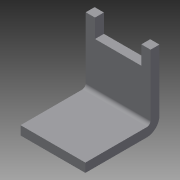
# Autodesk Inventor part: Glider
Saved by Autodesk Inventor 2013 (Build 170138000, 138)
## iProperties
Created: 2013-01-31
Part Number: Glider
Material: Generic
Document SubType Name: Sheet Metal
Designer: actoennies
Density: 1 g/cm^3
Sheet Metal Rule: Default
Author: actoennies
Autodesk Inventor part; units mm, degrees
ref_plane "YZ Plane" through (0, 0, 0) normal (1, 0, 0) x (0, 1, 0)
ref_plane "XZ Plane" through (0, 0, 0) normal (0, 1, 0) x (-1, 0, 0)
ref_plane "XY Plane" through (0, 0, 0) normal (0, 0, 1) x (1, 0, 0)
sketch "Sketch1" plane through (0, 0, 0) normal (0, 0, 1) x (1, 0, 0)
  line L0 (0, 0) -> (0, 6.35)
  line L1 (0, 6.35) -> (-3.175, 6.35)
  line L2 (-3.175, 6.35) -> (-3.175, -3.175)
  line L3 (0, 0) -> (15.875, 0)
  line L4 (15.875, 0) -> (15.875, 6.35)
  line L5 (15.875, 6.35) -> (19.05, 6.35)
  line L6 (19.05, 6.35) -> (19.05, -3.175)
  line L7 (-3.175, -3.175) -> (-3.175, -19.05)
  line L8 (-3.175, -19.05) -> (19.05, -19.05)
  line L9 (19.05, -19.05) -> (19.05, -3.175)
  dimension "d0" = 6.35
  dimension "d1" = 3.175
  dimension "d2" = 9.525
  dimension "d3" = 15.875
  dimension "d4" = 3.175
  dimension "d6" = 15.875
  measures "d0" distance of L0.start L0.end
  measures "d1" distance of L0.end L1.end
  measures "d2" distance of L1.end L2.end
  measures "d3" distance of L0.start L3.end
  measures "d4" distance of L4.end L5.end
  measures "d6" distance of L2.end L7.end
extrude "Plate1" add sketch "Sketch1" along normal blind 3.048
sketch "Sketch2" plane through (19.05, -16.002, 0) normal (0, -1, 0) x (1, 0, 0)
  line L0 (-22.225, 0) -> (0, 0)
  line L1 (0, 0) -> (0, 25.4)
  line L2 (0, 25.4) -> (-22.225, 25.4)
  line L3 (-22.225, 25.4) -> (-22.225, 0)
  constraints: 6 end point, 1 horizontal, 1 perpendicular, 1 vertical
edge flange "Flange1" height 25.4 angle 90 thickness 3.048 bend radius 1.27 thickness toward (0, -1, 0) relief tear relief width 3.048 relief depth 1.524 edges at (7.9375, -19.05, 3.048) wall of the first edge with corners at (-3.175, -16.002, 0) (19.05, -16.002, 0) (19.05, -16.002, 25.4) (-3.175, -16.002, 25.4)
bend "Bend1"
corner "Corner1"
sketch "Sketch3" plane through (-3.175, -16.002, 25.4) normal (0, 1, 0) x (1, 0, 0)
  line L0 (0, 0) -> (0, 21.082) projected
  line L1 (0, 0) -> (22.225, 0) projected
  line L2 (22.225, 0) -> (22.225, 21.082) projected
  circle A0 centre (6.35, 12.7) radius 3.3782
  circle A1 centre (15.875, 12.7) radius 3.3782
  point P0 (3.175, 25.4)
  dimension "d23" = 6.7564
  dimension "d24" = 6.7564
  dimension "d25" = 12.7
  dimension "d26" = 12.7
  dimension "d27" = 6.35
  dimension "d28" = 6.35
  constraints: 2 centre point
  measures "d23" diameter of A0
  measures "d24" diameter of A1
  measures "d25" distance from line of L1 A1.centre
  measures "d26" distance from line of L1 A0.centre
  measures "d27" distance from line of L2 A1.centre
  measures "d28" distance from line of L0 A0.centre
extrude "Cut1" cut sketch "Sketch3" against normal blind 3.048
equation "\"d29\" = Thickness"
equation "\"d13\" = BendReliefWidth"
equation "\"d14\" = BendReliefDepth"
equation "\"d15\" = MinimumRemnant"
equation "\"d16\" = BendRadius"
equation "\"d20\" = CornerReliefSize"
equation "\"d21\" = GapSize"
equation "\"d22\" = JacobiRadiusSize"
equation "\"BendRadius\" = Thickness"
equation "\"BendReliefWidth\" = Thickness"
equation "\"BendReliefDepth\" = 0.5 * Thickness"
equation "\"CornerReliefSize\" = 4 * Thickness"
equation "\"MinimumRemnant\" = 2 * Thickness"
equation "\"TransitionRadius\" = BendRadius"
equation "\"JacobiRadiusSize\" = BendRadius"
equation "\"GapSize\" = Thickness"
equation "\"d12\" = BendRadius"
equation "\"Thickness\" = 3.048"
body "Solid1"
